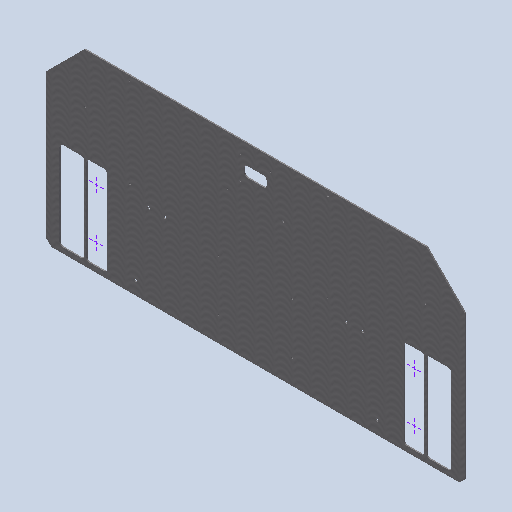
# Autodesk Inventor part: PlanchaBaseInferior
Saved by Autodesk Inventor 2022.1 (Build 261234000, 234)
## iProperties
Created: 2021-09-22
Part Number: PlanchaBaseInferior
Material: Steel, Mild, Welded
Document SubType Name: Sheet Metal
Designer: Andres
Density: 7.85 g/cm^3
Sheet Metal Rule: Por defecto_mm
Appearance: Weld - Steel Mild
Author: Andres
Autodesk Inventor part; units mm, degrees
ref_plane "YZ Plane" through (0, 0, 0) normal (1, 0, 0) x (0, 1, 0)
ref_plane "XZ Plane" through (0, 0, 0) normal (0, 1, 0) x (-1, 0, 0)
ref_plane "XY Plane" through (0, 0, 0) normal (0, 0, 1) x (1, 0, 0)
sketch "Sketch1" plane through (0, 0, 0) normal (0, 0, 1) x (1, 0, 0)
  line L0 (725.9853, -345.9853) -> (570.9853, -345.9853) construction
  line L1 (725.9853, -370.9853) -> (570.9853, -370.9853) construction
  line L2 (125.9853, -345.9853) -> (750.9853, -345.9853)
  line L3 (750.9853, -345.9853) -> (933.3076, -345.9853)
  line L4 (933.3076, -345.9853) -> (945.9853, -333.3076)
  line L5 (945.9853, -333.3076) -> (945.9853, 16.337)
  line L6 (945.9853, 16.337) -> (853.3076, 109.0147)
  line L7 (853.3076, 109.0147) -> (23.663, 109.0147)
  line L8 (-69.0147, 16.337) -> (23.663, 109.0147)
  line L9 (-69.0147, 16.337) -> (-69.0147, -333.3076)
  line L10 (-69.0147, -333.3076) -> (-56.337, -345.9853)
  line L11 (125.9853, -345.9853) -> (-56.337, -345.9853)
  line L12 (725.9853, -370.9853) -> (725.9853, -345.9853) projected
  line L13 (570.9853, -345.9853) -> (570.9853, -370.9853) projected
  constraints: 20 end point, 2 perpendicular, 1 collinear
extrude "Plate1" add sketch "Sketch1" along normal blind 3
sketch "Sketch2" plane through (0, 0, 0) normal (0, 0, 1) x (1, 0, 0)
  line L0 (-31.5147, -334.9853) -> (-31.5147, -114.9853) projected
  line L1 (18.4853, -114.9853) -> (18.4853, -334.9853) projected
  line L2 (33.4853, 101.5147) -> (33.4853, -338.4853) projected
  line L3 (73.4853, 101.5147) -> (73.4853, -338.4853) projected
  line L4 (803.4853, -338.4853) -> (803.4853, 101.5147) projected
  line L5 (843.4853, -338.4853) -> (843.4853, 101.5147) projected
  line L6 (858.4853, -334.9853) -> (858.4853, -114.9853) projected
  line L7 (908.4853, -114.9853) -> (908.4853, -334.9853) projected
  line L8 (860.9853, -327.9853) -> (905.9853, -327.9853)
  line L9 (908.4853, -325.4853) -> (908.4853, -125.4853)
  line L10 (905.9853, -122.9853) -> (860.9853, -122.9853)
  line L11 (858.4853, -125.4853) -> (858.4853, -325.4853)
  line L12 (-29.0147, -327.9853) -> (15.9853, -327.9853)
  line L13 (18.4853, -325.4853) -> (18.4853, -125.4853)
  line L14 (15.9853, -122.9853) -> (-29.0147, -122.9853)
  line L15 (-31.5147, -125.4853) -> (-31.5147, -325.4853)
  line L16 (-56.337, -345.9853) -> (933.3076, -345.9853) projected
  arc A0 (-31.5147, -325.4853) -> (-29.0147, -327.9853) centre (-29.0147, -325.4853) ccw
  arc A1 (15.9853, -327.9853) -> (18.4853, -325.4853) centre (15.9853, -325.4853) ccw
  arc A2 (18.4853, -125.4853) -> (15.9853, -122.9853) centre (15.9853, -125.4853) ccw
  arc A3 (-29.0147, -122.9853) -> (-31.5147, -125.4853) centre (-29.0147, -125.4853) ccw
  arc A4 (908.4853, -125.4853) -> (905.9853, -122.9853) centre (905.9853, -125.4853) ccw
  arc A5 (860.9853, -122.9853) -> (858.4853, -125.4853) centre (860.9853, -125.4853) ccw
  arc A6 (858.4853, -325.4853) -> (860.9853, -327.9853) centre (860.9853, -325.4853) ccw
  arc A7 (905.9853, -327.9853) -> (908.4853, -325.4853) centre (905.9853, -325.4853) ccw
  line L17 (905.9853, -332.9853) -> (860.9853, -332.9853)
  arc A8 (853.4853, -325.4853) -> (860.9853, -332.9853) centre (860.9853, -325.4853) ccw
  line L18 (853.4853, -325.4853) -> (853.4853, -125.4853)
  arc A9 (860.9853, -117.9853) -> (853.4853, -125.4853) centre (860.9853, -125.4853) ccw
  line L19 (860.9853, -117.9853) -> (905.9853, -117.9853)
  arc A10 (913.4853, -125.4853) -> (905.9853, -117.9853) centre (905.9853, -125.4853) ccw
  line L20 (913.4853, -125.4853) -> (913.4853, -325.4853)
  arc A11 (905.9853, -332.9853) -> (913.4853, -325.4853) centre (905.9853, -325.4853) ccw
  line L21 (15.9853, -332.9853) -> (-29.0147, -332.9853)
  arc A12 (-36.5147, -325.4853) -> (-29.0147, -332.9853) centre (-29.0147, -325.4853) ccw
  line L22 (-36.5147, -325.4853) -> (-36.5147, -125.4853)
  arc A13 (-29.0147, -117.9853) -> (-36.5147, -125.4853) centre (-29.0147, -125.4853) ccw
  line L23 (-29.0147, -117.9853) -> (15.9853, -117.9853)
  arc A14 (23.4853, -125.4853) -> (15.9853, -117.9853) centre (15.9853, -125.4853) ccw
  line L24 (23.4853, -125.4853) -> (23.4853, -325.4853)
  arc A15 (15.9853, -332.9853) -> (23.4853, -325.4853) centre (15.9853, -325.4853) ccw
  line L25 (35.9853, -327.9853) -> (70.9853, -327.9853)
  line L26 (73.4853, -325.4853) -> (73.4853, -125.4853)
  line L27 (70.9853, -122.9853) -> (35.9853, -122.9853)
  line L28 (33.4853, -125.4853) -> (33.4853, -325.4853)
  arc A16 (33.4853, -325.4853) -> (35.9853, -327.9853) centre (35.9853, -325.4853) ccw
  arc A17 (70.9853, -327.9853) -> (73.4853, -325.4853) centre (70.9853, -325.4853) ccw
  arc A18 (35.9853, -122.9853) -> (33.4853, -125.4853) centre (35.9853, -125.4853) ccw
  arc A19 (73.4853, -125.4853) -> (70.9853, -122.9853) centre (70.9853, -125.4853) ccw
  line L29 (70.9853, -332.9853) -> (35.9853, -332.9853)
  arc A20 (28.4853, -325.4853) -> (35.9853, -332.9853) centre (35.9853, -325.4853) ccw
  line L30 (28.4853, -325.4853) -> (28.4853, -125.4853)
  arc A21 (35.9853, -117.9853) -> (28.4853, -125.4853) centre (35.9853, -125.4853) ccw
  line L31 (35.9853, -117.9853) -> (70.9853, -117.9853)
  arc A22 (78.4853, -125.4853) -> (70.9853, -117.9853) centre (70.9853, -125.4853) ccw
  line L32 (78.4853, -125.4853) -> (78.4853, -325.4853)
  arc A23 (70.9853, -332.9853) -> (78.4853, -325.4853) centre (70.9853, -325.4853) ccw
  line L33 (15.9853, -332.9853) -> (35.9853, -332.9853)
  line L34 (15.9853, -117.9853) -> (35.9853, -117.9853)
  line L35 (805.9853, -327.9853) -> (840.9853, -327.9853)
  line L36 (843.4853, -325.4853) -> (843.4853, -125.4853)
  line L37 (840.9853, -122.9853) -> (805.9853, -122.9853)
  line L38 (803.4853, -125.4853) -> (803.4853, -325.4853)
  arc A24 (803.4853, -325.4853) -> (805.9853, -327.9853) centre (805.9853, -325.4853) ccw
  arc A25 (840.9853, -327.9853) -> (843.4853, -325.4853) centre (840.9853, -325.4853) ccw
  arc A26 (843.4853, -125.4853) -> (840.9853, -122.9853) centre (840.9853, -125.4853) ccw
  arc A27 (805.9853, -122.9853) -> (803.4853, -125.4853) centre (805.9853, -125.4853) ccw
  line L39 (840.9853, -332.9853) -> (805.9853, -332.9853)
  arc A28 (798.4853, -325.4853) -> (805.9853, -332.9853) centre (805.9853, -325.4853) ccw
  line L40 (798.4853, -325.4853) -> (798.4853, -125.4853)
  arc A29 (805.9853, -117.9853) -> (798.4853, -125.4853) centre (805.9853, -125.4853) ccw
  line L41 (805.9853, -117.9853) -> (840.9853, -117.9853)
  arc A30 (848.4853, -125.4853) -> (840.9853, -117.9853) centre (840.9853, -125.4853) ccw
  line L42 (848.4853, -125.4853) -> (848.4853, -325.4853)
  arc A31 (840.9853, -332.9853) -> (848.4853, -325.4853) centre (840.9853, -325.4853) ccw
  line L43 (840.9853, -332.9853) -> (860.9853, -332.9853)
  line L44 (840.9853, -117.9853) -> (860.9853, -117.9853)
  point P0 (438.4853, 79.5147)
  point P1 (858.4853, -327.9853)
  point P2 (908.4853, -122.9853)
  point P3 (-31.5147, -327.9853)
  point P4 (18.4853, -122.9853)
  point P5 (33.4853, -327.9853)
  point P6 (73.4853, -122.9853)
  point P7 (803.4853, -327.9853)
  point P8 (843.4853, -122.9853)
  dimension "d96" = 18
  dimension "d97" = 205
  dimension "d98" = 2.5
  dimension "d99" = 5
  dimension "d100" = 5
  dimension "d101" = 2.5
  dimension "d102" = 5
  dimension "d103" = 2.5
  dimension "d104" = 5
  constraints: 72 end point, 64 point on circle, 33 tangent, 32 centre point, 27 point on line, 16 parallel, 13 equal radius, 8 perpendicular, 5 collinear, 4 horizontal, 28 other
  measures "d96" distance between parallel lines of L16 L12
  measures "d97" distance between parallel lines of L14 L12
  measures "d98" radius of A0
  measures "d99" distance between parallel lines of L8 L17
  measures "d100" distance between parallel lines of L12 L21
  measures "d101" radius of A16
  measures "d102" distance between parallel lines of L25 L29
  measures "d103" radius of A24
  measures "d104" distance between parallel lines of L35 L39
extrude "Cut1" cut sketch "Sketch2" along normal through all contours L0 A12 L22 A13 | A0 L12 A1 L1 A15 L21 A12 L0 | L0 A3 L14 A2 L1 A1 L12 A0 | L0 A13 L23 A14 L1 A2 L14 A3 | L1 A14 L24 A15 | A20 L30 A21 L2 | L2 A16 L25 A17 L3 A23 L29 A20 | A21 L31 A22 L3 A19 L27 A18 L2 | L2 A18 L27 A19 L3 A17 L25 A16 | L3 A22 L32 A23 | L4 A28 L40 A29 | A24 L35 A25 L5 A31 L39 A28 L4 | L4 A27 L37 A26 L5 A25 L35 A24 | L4 A29 L41 A30 L5 A26 L37 A27 | L5 A30 L42 A31 | A8 L18 A9 L6 | L6 A6 L8 A7 L7 A11 L17 A8 | A9 L19 A10 L7 A4 L10 A5 L6 | L6 A5 L10 A4 L7 A7 L8 A6 | L7 A10 L20 A11
sketch "Sketch4" plane through (0, 0, 3) normal (0, 0, 1) x (1, 0, 0)
  line L0 (933.3076, -345.9853) -> (-56.337, -345.9853) projected
  line L1 (-56.337, -345.9853) -> (933.3076, -345.9853) construction
  line L2 (438.4853, 109.0147) -> (438.4853, 49.0147) construction
  line L3 (401.4853, 21.0147) -> (475.4853, 21.0147) construction
  line L4 (475.4853, 21.0147) -> (475.4853, 77.0147) construction
  line L5 (475.4853, 77.0147) -> (401.4853, 77.0147) construction
  line L6 (401.4853, 77.0147) -> (401.4853, 21.0147) construction
  line L7 (401.4853, 21.0147) -> (475.4853, 77.0147) construction
  line L8 (475.4853, 21.0147) -> (401.4853, 77.0147) construction
  line L9 (411.4853, 36.5147) -> (465.4853, 36.5147)
  line L10 (465.4853, 36.5147) -> (465.4853, 61.5147)
  line L11 (465.4853, 61.5147) -> (411.4853, 61.5147)
  line L12 (411.4853, 61.5147) -> (411.4853, 36.5147)
  line L13 (411.4853, 36.5147) -> (465.4853, 61.5147) construction
  line L14 (465.4853, 36.5147) -> (411.4853, 61.5147) construction
  line L15 (23.663, 109.0147) -> (853.3076, 109.0147) projected
  point P0 (0, 0)
  dimension "d46" = 74
  dimension "d47" = 56
  dimension "d55" = 54
  dimension "d56" = 25
  dimension "d59" = 60
  constraints: 26 end point, 5 midpoint, 4 coincident, 4 parallel, 2 horizontal, 2 perpendicular, 1 vertical
  measures "d46" distance of L5.end L4.end
  measures "d47" distance of L4.end L3.end
  measures "d55" distance between parallel lines of L10 L12
  measures "d56" distance between parallel lines of L11 L9
  measures "d59" distance of L2.start L2.end
hole "Hole1" at (401.4853, 77.0147, 3) at (401.4853, 21.0147, 3) at (475.4853, 21.0147, 3) at (475.4853, 77.0147, 3) direction (0, 0, -1) diameter 3.4 end through all clearance for "Countersunk Flat Head Screw ISO 2009/7046" size "M3" standard "ISO"
extrude "Cut3" cut sketch "Sketch4" against normal blind 3
fillet "Corner Round2" radius 6 4 edges at (411.4853, 61.5147, 1.5) (411.4853, 36.5147, 1.5) (465.4853, 61.5147, 1.5) (465.4853, 36.5147, 1.5)
sketch "Sketch5" plane through (0, 0, 3) normal (0, 0, 1) x (1, 0, 0)
  circle A0 centre (219.1853, -146.4853) radius 3.3 projected
  circle A1 centre (179.1853, -146.4853) radius 3.3 projected
  circle A2 centre (147.6853, -314.4853) radius 3.3 projected
  circle A3 centre (349.1853, -162.9853) radius 3 projected
  circle A4 centre (349.1853, -286.9853) radius 2.2 projected
  arc A5 (34.2552, -163.466) -> (33.5853, -165.966) centre (38.5853, -165.966) ccw projected
  line L0 (33.5853, -175.2353) -> (33.5853, -165.966) projected
  line L1 (73.5853, -175.2353) -> (33.5853, -175.2353) projected
  arc A6 (48.0853, -167.9853) -> (59.0853, -167.9853) centre (53.5853, -167.9853) ccw projected
  line L2 (48.0853, -167.9853) -> (48.0853, -160.9853) projected
  arc A7 (59.0853, -160.9853) -> (48.0853, -160.9853) centre (53.5853, -160.9853) ccw projected
  line L3 (59.0853, -160.9853) -> (59.0853, -167.9853) projected
  line L4 (73.5853, -165.966) -> (73.5853, -175.2353) projected
  arc A8 (73.5853, -165.966) -> (72.9154, -163.466) centre (68.5853, -165.966) ccw projected
  line L5 (72.9154, -163.466) -> (67.0087, -153.2353) projected
  arc A9 (67.0087, -153.2353) -> (40.1619, -153.2353) centre (53.5853, -160.9853) ccw projected
  line L6 (40.1619, -153.2353) -> (34.2552, -163.466) projected
  arc A10 (33.5853, -284.0045) -> (34.2552, -286.5045) centre (38.5853, -284.0045) ccw projected
  line L7 (34.2552, -286.5045) -> (40.1619, -296.7353) projected
  arc A11 (40.1619, -296.7353) -> (67.0087, -296.7353) centre (53.5853, -288.9853) ccw projected
  line L8 (67.0087, -296.7353) -> (72.9154, -286.5045) projected
  arc A12 (72.9154, -286.5045) -> (73.5853, -284.0045) centre (68.5853, -284.0045) ccw projected
  line L9 (73.5853, -274.7353) -> (73.5853, -284.0045) projected
  line L10 (73.5853, -274.7353) -> (33.5853, -274.7353) projected
  arc A13 (59.0853, -281.9853) -> (48.0853, -281.9853) centre (53.5853, -281.9853) ccw projected
  line L11 (59.0853, -281.9853) -> (59.0853, -288.9853) projected
  arc A14 (48.0853, -288.9853) -> (59.0853, -288.9853) centre (53.5853, -288.9853) ccw projected
  line L12 (48.0853, -288.9853) -> (48.0853, -281.9853) projected
  line L13 (33.5853, -284.0045) -> (33.5853, -274.7353) projected
  circle A15 centre (527.7853, -162.9853) radius 2.2 projected
  circle A16 centre (527.7853, -286.9853) radius 3 projected
  arc A17 (843.3853, -165.966) -> (842.7154, -163.466) centre (838.3853, -165.966) ccw projected
  line L14 (842.7154, -163.466) -> (836.8087, -153.2353) projected
  arc A18 (836.8087, -153.2353) -> (809.9619, -153.2353) centre (823.3853, -160.9853) ccw projected
  line L15 (809.9619, -153.2353) -> (804.0552, -163.466) projected
  arc A19 (804.0552, -163.466) -> (803.3853, -165.966) centre (808.3853, -165.966) ccw projected
  line L16 (803.3853, -175.2353) -> (803.3853, -165.966) projected
  line L17 (803.3853, -175.2353) -> (843.3853, -175.2353) projected
  arc A20 (817.8853, -167.9853) -> (828.8853, -167.9853) centre (823.3853, -167.9853) ccw projected
  line L18 (817.8853, -167.9853) -> (817.8853, -160.9853) projected
  arc A21 (828.8853, -160.9853) -> (817.8853, -160.9853) centre (823.3853, -160.9853) ccw projected
  line L19 (828.8853, -160.9853) -> (828.8853, -167.9853) projected
  line L20 (843.3853, -165.966) -> (843.3853, -175.2353) projected
  arc A22 (842.7154, -286.5045) -> (843.3853, -284.0045) centre (838.3853, -284.0045) ccw projected
  line L21 (843.3853, -274.7353) -> (843.3853, -284.0045) projected
  line L22 (803.3853, -274.7353) -> (843.3853, -274.7353) projected
  arc A23 (828.8853, -281.9853) -> (817.8853, -281.9853) centre (823.3853, -281.9853) ccw projected
  line L23 (828.8853, -281.9853) -> (828.8853, -288.9853) projected
  arc A24 (817.8853, -288.9853) -> (828.8853, -288.9853) centre (823.3853, -288.9853) ccw projected
  line L24 (817.8853, -288.9853) -> (817.8853, -281.9853) projected
  line L25 (803.3853, -284.0045) -> (803.3853, -274.7353) projected
  arc A25 (803.3853, -284.0045) -> (804.0552, -286.5045) centre (808.3853, -284.0045) ccw projected
  line L26 (804.0552, -286.5045) -> (809.9619, -296.7353) projected
  arc A26 (809.9619, -296.7353) -> (836.8087, -296.7353) centre (823.3853, -288.9853) ccw projected
  line L27 (836.8087, -296.7353) -> (842.7154, -286.5045) projected
  circle A27 centre (697.7853, -146.4853) radius 3.3 projected
  circle A28 centre (657.7853, -146.4853) radius 3.3 projected
  circle A29 centre (733.7853, -314.4853) radius 3.3 projected
  point P0 (0, 0)
sketch "Sketch6" plane through (0, 0, 0) normal (0, 0, -1) x (-1, 0, 0)
  point P0 (-657.7853, -146.4853)
  point P1 (-697.7853, -146.4853)
  point P2 (-219.1853, -146.4853)
  point P3 (-179.1853, -146.4853)
  point P4 (-733.7853, -314.4853)
  point P5 (-147.6853, -314.4853)
hole "Hole2" at (657.7853, -146.4853, 0) at (697.7853, -146.4853, 0) at (219.1853, -146.4853, 0) at (179.1853, -146.4853, 0) at (733.7853, -314.4853, 0) at (147.6853, -314.4853, 0) direction (0, 0, 1) diameter 6.6 end through all
sketch "Sketch7" plane through (0, 0, 0) normal (0, 0, -1) x (-1, 0, 0)
  point P0 (-527.7853, -162.9853)
  point P1 (-527.7853, -286.9853)
  point P2 (-349.1853, -286.9853)
  point P3 (-349.1853, -162.9853)
hole "Hole3" at (527.7853, -162.9853, 0) at (527.7853, -286.9853, 0) at (349.1853, -286.9853, 0) at (349.1853, -162.9853, 0) direction (0, 0, 1) diameter 4.5 end through all
sketch "Sketch9" plane through (0, 0, 3) normal (0, 0, 1) x (1, 0, 0)
  point P0 (53.5853, -160.9853)
  point P1 (53.5853, -281.9853)
  point P2 (823.3853, -160.9853)
  point P3 (823.3853, -281.9853)
sketch "Sketch10" plane through (0, 0, 0) normal (0, 0, -1) x (-1, 0, 0)
  point P0 (-613.8153, 96.5147)
  point P1 (-851.1853, -11.3153)
  point P2 (-505.9853, -11.3153)
  point P3 (-370.9853, -11.3153)
  point P4 (-133.6153, 96.5147)
  point P5 (-133.6153, -119.1453)
  point P6 (-25.7853, -11.3153)
  point P7 (-613.8153, -119.1453)
hole "Hole6" at (613.8153, 96.5147, 0) at (851.1853, -11.3153, 0) at (505.9853, -11.3153, 0) at (370.9853, -11.3153, 0) at (133.6153, 96.5147, 0) at (133.6153, -119.1453, 0) at (25.7853, -11.3153, 0) at (613.8153, -119.1453, 0) direction (0, 0, 1) diameter 4.5 end through all
equation "\"d6\" = Thickness"
equation "\"d53\" = Thickness"
equation "\"d57\" = Thickness"
equation "\"d0\" = Thickness"
equation "\"BendRadius\" = Thickness"
equation "\"BendReliefWidth\" = Thickness"
equation "\"BendReliefDepth\" = 0.5 * Thickness"
equation "\"CornerReliefSize\" = 4 * Thickness"
equation "\"MinimumRemnant\" = 2 * Thickness"
equation "\"TransitionRadius\" = BendRadius"
equation "\"JacobiRadiusSize\" = BendRadius"
equation "\"GapSize\" = Thickness"
equation "\"Thickness\" = 3"
body "Solid1"
